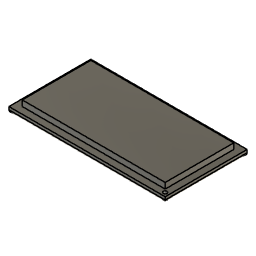
controller lid (Autodesk Fusion 360 design; units mm, degrees)
Autodesk Fusion 360 part; units mm, degrees
sketch "Sketch1" plane through (0, 0, 0) normal (0, 0, 1) x (1, 0, 0)
  line L0 (0, 0) -> (82, 0)
  line L1 (82, 0) -> (82, 43)
  line L2 (82, 43) -> (0, 43)
  line L3 (0, 43) -> (0, 0)
  dimension "d1" = 82
  dimension "d2" = 43
  constraint horizontal L0
  constraint vertical L1
  constraint horizontal L2
  constraint vertical L3
  constraint coincident L0.start L3.end
  measures "d1" distance of L0.start L0.end
  measures "d2" distance of L0.start L2.end
extrude "Extrude1" add sketch "Sketch1" along normal blind 3
sketch "Sketch2" plane through (0, 0, 3) normal (0, 0, 1) x (-1, 0, 0)
  line L0 (0, -43) -> (0, 0)
  line L1 (0, 0) -> (-82, 0)
  line L2 (-82, 0) -> (-82, -43)
  line L3 (-82, -43) -> (0, -43)
  line L4 (-3.5, -3.5) -> (-78.5, -3.5)
  line L5 (-78.5, -3.5) -> (-78.5, -39.5)
  line L6 (-78.5, -39.5) -> (-3.5, -39.5)
  line L7 (-3.5, -39.5) -> (-3.5, -3.5)
  dimension "d5" = 3.5
  dimension "d6" = 3.5
  dimension "d7" = 3.5
  dimension "d8" = 3.5
  constraint horizontal L4
  constraint vertical L5
  constraint horizontal L6
  constraint vertical L7
  measures "d5" distance of L1 L4
  measures "d6" distance of L3 L6
  measures "d7" distance of L0 L7
  measures "d8" distance of L2 L5
extrude "Extrude2" add sketch "Sketch2" along normal blind 3 contours L4 L5 L6 L7
sketch "Sketch4" plane through (0, 0, 0) normal (0, 0, -1) x (1, 0, 0)
  line L0 (0, 0) -> (0, -43)
  line L1 (0, -43) -> (82, -43)
  line L2 (82, -43) -> (82, 0)
  line L3 (82, 0) -> (0, 0)
  circle A0 centre (2, -41) radius 1
  circle A1 centre (80, -2) radius 1
  dimension "d14" = 2
  dimension "d15" = 2
  dimension "d16" = 2
  dimension "d17" = 2
  dimension "d18" = 2
  dimension "d19" = 2
  measures "d14" diameter of A0
  measures "d15" distance of L1 A0.centre
  measures "d16" distance of L0 A0.centre
  measures "d17" diameter of A1
  measures "d18" distance of L3 A1.centre
  measures "d19" distance of L2 A1.centre
extrude "Extrude3" cut sketch "Sketch4" against normal blind 3 contours A0 | A1
fillet "Fillet2" radius 1.5 4 edges at (0, 21.5, 0) (41, 43, 0) (41, 0, 0) (82, 21.5, 0)
